calf_dyno_enclosure (Autodesk Fusion 360 design; units mm, degrees)
Autodesk Fusion 360 part; units mm, degrees
sketch "Outer shell blank profile" plane through (0, 0, 0) normal (0, 0, 1) x (1, 0, 0) in component "Base - print floor down"
  line L0 (10, 10) -> (100, 10)
  line L1 (100, 10) -> (100, 75)
  line L2 (100, 75) -> (10, 75)
  line L3 (10, 75) -> (10, 10)
  dimension "d23" = 10
  dimension "d24" = 10
  dimension "d25" = 90
  dimension "d26" = 65
  measures "d23" horizontal distance of origin L0.start
  measures "d24" vertical distance of origin L0.start
  measures "d25" horizontal distance of L0.start L0.end
  measures "d26" vertical distance of L0.end L1.end
extrude "Outer shell blank" add sketch "Outer shell blank profile" along normal blind 32 makes body 1 in component "Base - print floor down"
fillet "Rounded outside corners" radius 2 4 edges at (10, 75, 16) (100, 75, 16) (100, 10, 16) (10, 10, 16) on bodies 1 in component "Base - print floor down"
sketch "Electronics cavity profile" plane through (0, 0, 0) normal (0, 0, 1) x (1, 0, 0) in component "Base - print floor down"
  line L0 (12, 12) -> (98, 12)
  line L1 (98, 12) -> (98, 73)
  line L2 (98, 73) -> (12, 73)
  line L3 (12, 73) -> (12, 12)
  dimension "d32" = 12
  dimension "d33" = 12
  dimension "d34" = 86
  dimension "d35" = 61
  measures "d32" horizontal distance of origin L0.start
  measures "d33" vertical distance of origin L0.start
  measures "d34" horizontal distance of L0.start L0.end
  measures "d35" vertical distance of L0.end L1.end
extrude "Electronics cavity" cut sketch "Electronics cavity profile" along normal blind 31 from surface at 2 bodies 1 in component "Base - print floor down"
sketch "USB-C plug access profile" plane through (0, 0, 0) normal (0, 0, 1) x (1, 0, 0) in component "Base - print floor down"
  line L0 (9, 34.5) -> (13, 34.5)
  line L1 (13, 34.5) -> (13, 50.5)
  line L2 (13, 50.5) -> (9, 50.5)
  line L3 (9, 50.5) -> (9, 34.5)
  dimension "d39" = 9
  dimension "d40" = 34.5
  dimension "d41" = 4
  dimension "d42" = 16
  measures "d39" horizontal distance of origin L0.start
  measures "d40" vertical distance of origin L0.start
  measures "d41" horizontal distance of L0.start L0.end
  measures "d42" vertical distance of L0.end L1.end
extrude "USB-C plug access" cut sketch "USB-C plug access profile" along normal blind 10 from surface at 4 bodies 1 in component "Base - print floor down"
sketch "Drop-in load-cell cable notch profile" plane through (0, 0, 0) normal (0, 0, 1) x (1, 0, 0) in component "Base - print floor down"
  line L0 (97, 39) -> (101, 39)
  line L1 (101, 39) -> (101, 46)
  line L2 (101, 46) -> (97, 46)
  line L3 (97, 46) -> (97, 39)
  dimension "d46" = 97
  dimension "d47" = 39
  dimension "d48" = 4
  dimension "d49" = 7
  measures "d46" horizontal distance of origin L0.start
  measures "d47" vertical distance of origin L0.start
  measures "d48" horizontal distance of L0.start L0.end
  measures "d49" vertical distance of L0.end L1.end
extrude "Drop-in load-cell cable notch" cut sketch "Drop-in load-cell cable notch profile" along normal blind 8 from surface at 25 bodies 1 in component "Base - print floor down"
fillet "Rounded cable seat" radius 3.3 2 edges at (99, 39, 25) (99, 46, 25) on bodies 1 in component "Base - print floor down"
sketch "Snap window front outer_length * 0.23 profile" plane through (0, 0, 0) normal (0, 0, 1) x (1, 0, 0) in component "Base - print floor down"
  line L0 (26.4, 9) -> (35, 9)
  line L1 (35, 9) -> (35, 13)
  line L2 (35, 13) -> (26.4, 13)
  line L3 (26.4, 13) -> (26.4, 9)
  dimension "d55" = 26.4
  dimension "d56" = 9
  dimension "d57" = 8.6
  dimension "d58" = 4
  measures "d55" horizontal distance of origin L0.start
  measures "d56" vertical distance of origin L0.start
  measures "d57" horizontal distance of L0.start L0.end
  measures "d58" vertical distance of L0.end L1.end
extrude "Snap window front outer_length * 0.23" cut sketch "Snap window front outer_length * 0.23 profile" along normal blind 2.6 from surface at 17.7 bodies 1 in component "Base - print floor down"
sketch "Snap window back outer_length * 0.23 profile" plane through (0, 0, 0) normal (0, 0, 1) x (1, 0, 0) in component "Base - print floor down"
  line L0 (26.4, 72) -> (35, 72)
  line L1 (35, 72) -> (35, 76)
  line L2 (35, 76) -> (26.4, 76)
  line L3 (26.4, 76) -> (26.4, 72)
  dimension "d62" = 26.4
  dimension "d63" = 72
  dimension "d64" = 8.6
  dimension "d65" = 4
  measures "d62" horizontal distance of origin L0.start
  measures "d63" vertical distance of origin L0.start
  measures "d64" horizontal distance of L0.start L0.end
  measures "d65" vertical distance of L0.end L1.end
extrude "Snap window back outer_length * 0.23" cut sketch "Snap window back outer_length * 0.23 profile" along normal blind 2.6 from surface at 17.7 bodies 1 in component "Base - print floor down"
sketch "Snap window front outer_length * 0.77 profile" plane through (0, 0, 0) normal (0, 0, 1) x (1, 0, 0) in component "Base - print floor down"
  line L0 (75, 9) -> (83.6, 9)
  line L1 (83.6, 9) -> (83.6, 13)
  line L2 (83.6, 13) -> (75, 13)
  line L3 (75, 13) -> (75, 9)
  dimension "d69" = 75
  dimension "d70" = 9
  dimension "d71" = 8.6
  dimension "d72" = 4
  measures "d69" horizontal distance of origin L0.start
  measures "d70" vertical distance of origin L0.start
  measures "d71" horizontal distance of L0.start L0.end
  measures "d72" vertical distance of L0.end L1.end
extrude "Snap window front outer_length * 0.77" cut sketch "Snap window front outer_length * 0.77 profile" along normal blind 2.6 from surface at 17.7 bodies 1 in component "Base - print floor down"
sketch "Snap window back outer_length * 0.77 profile" plane through (0, 0, 0) normal (0, 0, 1) x (1, 0, 0) in component "Base - print floor down"
  line L0 (75, 72) -> (83.6, 72)
  line L1 (83.6, 72) -> (83.6, 76)
  line L2 (83.6, 76) -> (75, 76)
  line L3 (75, 76) -> (75, 72)
  dimension "d76" = 75
  dimension "d77" = 72
  dimension "d78" = 8.6
  dimension "d79" = 4
  measures "d76" horizontal distance of origin L0.start
  measures "d77" vertical distance of origin L0.start
  measures "d78" horizontal distance of L0.start L0.end
  measures "d79" vertical distance of L0.end L1.end
extrude "Snap window back outer_length * 0.77" cut sketch "Snap window back outer_length * 0.77 profile" along normal blind 2.6 from surface at 17.7 bodies 1 in component "Base - print floor down"
sketch "Cable tie anchor profile" plane through (0, 0, 0) normal (0, 0, 1) x (1, 0, 0) in component "Base - print floor down"
  line L0 (84, 37.5) -> (92, 37.5)
  line L1 (92, 37.5) -> (92, 47.5)
  line L2 (92, 47.5) -> (84, 47.5)
  line L3 (84, 47.5) -> (84, 37.5)
  dimension "d83" = 84
  dimension "d84" = 37.5
  dimension "d85" = 8
  dimension "d86" = 10
  measures "d83" horizontal distance of origin L0.start
  measures "d84" vertical distance of origin L0.start
  measures "d85" horizontal distance of L0.start L0.end
  measures "d86" vertical distance of L0.end L1.end
extrude "Cable tie anchor" add sketch "Cable tie anchor profile" along normal blind 5 from surface at 2 bodies 1 in component "Base - print floor down"
sketch "Cable tie tunnel profile" plane through (0, 0, 0) normal (0, 0, 1) x (1, 0, 0) in component "Base - print floor down"
  line L0 (83, 40.5) -> (93, 40.5)
  line L1 (93, 40.5) -> (93, 44.5)
  line L2 (93, 44.5) -> (83, 44.5)
  line L3 (83, 44.5) -> (83, 40.5)
  dimension "d90" = 83
  dimension "d91" = 40.5
  dimension "d92" = 10
  dimension "d93" = 4
  measures "d90" horizontal distance of origin L0.start
  measures "d91" vertical distance of origin L0.start
  measures "d92" horizontal distance of L0.start L0.end
  measures "d93" vertical distance of L0.end L1.end
extrude "Cable tie tunnel" cut sketch "Cable tie tunnel profile" along normal blind 2 from surface at 3 bodies 1 in component "Base - print floor down"
sketch "Lid plate profile" plane through (0, 0, 0) normal (0, 0, 1) x (1, 0, 0) in component "Lid - print outside face down"
  line L0 (10, 10) -> (100, 10)
  line L1 (100, 10) -> (100, 75)
  line L2 (100, 75) -> (10, 75)
  line L3 (10, 75) -> (10, 10)
  dimension "d97" = 10
  dimension "d98" = 10
  dimension "d99" = 90
  dimension "d100" = 65
  measures "d97" horizontal distance of origin L0.start
  measures "d98" vertical distance of origin L0.start
  measures "d99" horizontal distance of L0.start L0.end
  measures "d100" vertical distance of L0.end L1.end
extrude "Lid plate" add sketch "Lid plate profile" along normal blind 2 from surface at 32 separate body makes body 2 in component "Lid - print outside face down"
fillet "Lid outside corners" radius 2 4 edges at (10, 75, 33) (100, 75, 33) (100, 10, 33) (10, 10, 33) on bodies 2 in component "Lid - print outside face down"
sketch "Guide left front profile" plane through (0, 0, 0) normal (0, 0, 1) x (1, 0, 0) in component "Lid - print outside face down"
  line L0 (12.3, 12.3) -> (19.3, 12.3)
  line L1 (19.3, 12.3) -> (19.3, 13.5)
  line L2 (19.3, 13.5) -> (12.3, 13.5)
  line L3 (12.3, 13.5) -> (12.3, 12.3)
  dimension "d106" = 12.3
  dimension "d107" = 12.3
  dimension "d108" = 7
  dimension "d109" = 1.2
  measures "d106" horizontal distance of origin L0.start
  measures "d107" vertical distance of origin L0.start
  measures "d108" horizontal distance of L0.start L0.end
  measures "d109" vertical distance of L0.end L1.end
extrude "Guide left front" add sketch "Guide left front profile" along normal blind 3 from surface at 29 bodies 2 in component "Lid - print outside face down"
sketch "Guide left back profile" plane through (0, 0, 0) normal (0, 0, 1) x (1, 0, 0) in component "Lid - print outside face down"
  line L0 (12.3, 71.5) -> (19.3, 71.5)
  line L1 (19.3, 71.5) -> (19.3, 72.7)
  line L2 (19.3, 72.7) -> (12.3, 72.7)
  line L3 (12.3, 72.7) -> (12.3, 71.5)
  dimension "d113" = 12.3
  dimension "d114" = 71.5
  dimension "d115" = 7
  dimension "d116" = 1.2
  measures "d113" horizontal distance of origin L0.start
  measures "d114" vertical distance of origin L0.start
  measures "d115" horizontal distance of L0.start L0.end
  measures "d116" vertical distance of L0.end L1.end
extrude "Guide left back" add sketch "Guide left back profile" along normal blind 3 from surface at 29 bodies 2 in component "Lid - print outside face down"
sketch "Guide right front profile" plane through (0, 0, 0) normal (0, 0, 1) x (1, 0, 0) in component "Lid - print outside face down"
  line L0 (90.7, 12.3) -> (97.7, 12.3)
  line L1 (97.7, 12.3) -> (97.7, 13.5)
  line L2 (97.7, 13.5) -> (90.7, 13.5)
  line L3 (90.7, 13.5) -> (90.7, 12.3)
  dimension "d120" = 90.7
  dimension "d121" = 12.3
  dimension "d122" = 7
  dimension "d123" = 1.2
  measures "d120" horizontal distance of origin L0.start
  measures "d121" vertical distance of origin L0.start
  measures "d122" horizontal distance of L0.start L0.end
  measures "d123" vertical distance of L0.end L1.end
extrude "Guide right front" add sketch "Guide right front profile" along normal blind 3 from surface at 29 bodies 2 in component "Lid - print outside face down"
sketch "Guide right back profile" plane through (0, 0, 0) normal (0, 0, 1) x (1, 0, 0) in component "Lid - print outside face down"
  line L0 (90.7, 71.5) -> (97.7, 71.5)
  line L1 (97.7, 71.5) -> (97.7, 72.7)
  line L2 (97.7, 72.7) -> (90.7, 72.7)
  line L3 (90.7, 72.7) -> (90.7, 71.5)
  dimension "d127" = 90.7
  dimension "d128" = 71.5
  dimension "d129" = 7
  dimension "d130" = 1.2
  measures "d127" horizontal distance of origin L0.start
  measures "d128" vertical distance of origin L0.start
  measures "d129" horizontal distance of L0.start L0.end
  measures "d130" vertical distance of L0.end L1.end
extrude "Guide right back" add sketch "Guide right back profile" along normal blind 3 from surface at 29 bodies 2 in component "Lid - print outside face down"
sketch "End guide left front profile" plane through (0, 0, 0) normal (0, 0, 1) x (1, 0, 0) in component "Lid - print outside face down"
  line L0 (12.3, 12.3) -> (13.5, 12.3)
  line L1 (13.5, 12.3) -> (13.5, 19.3)
  line L2 (13.5, 19.3) -> (12.3, 19.3)
  line L3 (12.3, 19.3) -> (12.3, 12.3)
  dimension "d134" = 12.3
  dimension "d135" = 12.3
  dimension "d136" = 1.2
  dimension "d137" = 7
  measures "d134" horizontal distance of origin L0.start
  measures "d135" vertical distance of origin L0.start
  measures "d136" horizontal distance of L0.start L0.end
  measures "d137" vertical distance of L0.end L1.end
extrude "End guide left front" add sketch "End guide left front profile" along normal blind 3 from surface at 29 bodies 2 in component "Lid - print outside face down"
sketch "End guide left back profile" plane through (0, 0, 0) normal (0, 0, 1) x (1, 0, 0) in component "Lid - print outside face down"
  line L0 (12.3, 65.7) -> (13.5, 65.7)
  line L1 (13.5, 65.7) -> (13.5, 72.7)
  line L2 (13.5, 72.7) -> (12.3, 72.7)
  line L3 (12.3, 72.7) -> (12.3, 65.7)
  dimension "d141" = 12.3
  dimension "d142" = 65.7
  dimension "d143" = 1.2
  dimension "d144" = 7
  measures "d141" horizontal distance of origin L0.start
  measures "d142" vertical distance of origin L0.start
  measures "d143" horizontal distance of L0.start L0.end
  measures "d144" vertical distance of L0.end L1.end
extrude "End guide left back" add sketch "End guide left back profile" along normal blind 3 from surface at 29 bodies 2 in component "Lid - print outside face down"
sketch "End guide right front profile" plane through (0, 0, 0) normal (0, 0, 1) x (1, 0, 0) in component "Lid - print outside face down"
  line L0 (96.5, 12.3) -> (97.7, 12.3)
  line L1 (97.7, 12.3) -> (97.7, 19.3)
  line L2 (97.7, 19.3) -> (96.5, 19.3)
  line L3 (96.5, 19.3) -> (96.5, 12.3)
  dimension "d148" = 96.5
  dimension "d149" = 12.3
  dimension "d150" = 1.2
  dimension "d151" = 7
  measures "d148" horizontal distance of origin L0.start
  measures "d149" vertical distance of origin L0.start
  measures "d150" horizontal distance of L0.start L0.end
  measures "d151" vertical distance of L0.end L1.end
extrude "End guide right front" add sketch "End guide right front profile" along normal blind 3 from surface at 29 bodies 2 in component "Lid - print outside face down"
sketch "End guide right back profile" plane through (0, 0, 0) normal (0, 0, 1) x (1, 0, 0) in component "Lid - print outside face down"
  line L0 (96.5, 65.7) -> (97.7, 65.7)
  line L1 (97.7, 65.7) -> (97.7, 72.7)
  line L2 (97.7, 72.7) -> (96.5, 72.7)
  line L3 (96.5, 72.7) -> (96.5, 65.7)
  dimension "d155" = 96.5
  dimension "d156" = 65.7
  dimension "d157" = 1.2
  dimension "d158" = 7
  measures "d155" horizontal distance of origin L0.start
  measures "d156" vertical distance of origin L0.start
  measures "d157" horizontal distance of L0.start L0.end
  measures "d158" vertical distance of L0.end L1.end
extrude "End guide right back" add sketch "End guide right back profile" along normal blind 3 from surface at 29 bodies 2 in component "Lid - print outside face down"
sketch "Flexible snap front0 profile" plane through (0, 0, 0) normal (0, 0, 1) x (1, 0, 0) in component "Lid - print outside face down"
  line L0 (26.7, 12.3) -> (34.7, 12.3)
  line L1 (34.7, 12.3) -> (34.7, 13.5)
  line L2 (34.7, 13.5) -> (26.7, 13.5)
  line L3 (26.7, 13.5) -> (26.7, 12.3)
  dimension "d162" = 26.7
  dimension "d163" = 12.3
  dimension "d164" = 8
  dimension "d165" = 1.2
  measures "d162" horizontal distance of origin L0.start
  measures "d163" vertical distance of origin L0.start
  measures "d164" horizontal distance of L0.start L0.end
  measures "d165" vertical distance of L0.end L1.end
extrude "Flexible snap front0" add sketch "Flexible snap front0 profile" along normal blind 14 from surface at 18 bodies 2 in component "Lid - print outside face down"
sketch "Snap hook front0 profile" plane through (0, 0, 0) normal (0, 0, 1) x (1, 0, 0) in component "Lid - print outside face down"
  line L0 (26.7, 11.75) -> (34.7, 11.75)
  line L1 (34.7, 11.75) -> (34.7, 13.5)
  line L2 (34.7, 13.5) -> (26.7, 13.5)
  line L3 (26.7, 13.5) -> (26.7, 11.75)
  dimension "d169" = 26.7
  dimension "d170" = 11.75
  dimension "d171" = 8
  dimension "d172" = 1.75
  measures "d169" horizontal distance of origin L0.start
  measures "d170" vertical distance of origin L0.start
  measures "d171" horizontal distance of L0.start L0.end
  measures "d172" vertical distance of L0.end L1.end
extrude "Snap hook front0" add sketch "Snap hook front0 profile" along normal blind 2 from surface at 18 bodies 2 in component "Lid - print outside face down"
chamfer "Insertion ramp front0" distance 0.55 angle 45 1 edges at (30.7, 11.75, 18) on bodies 2 in component "Lid - print outside face down"
sketch "Flexible snap back0 profile" plane through (0, 0, 0) normal (0, 0, 1) x (1, 0, 0) in component "Lid - print outside face down"
  line L0 (26.7, 71.5) -> (34.7, 71.5)
  line L1 (34.7, 71.5) -> (34.7, 72.7)
  line L2 (34.7, 72.7) -> (26.7, 72.7)
  line L3 (26.7, 72.7) -> (26.7, 71.5)
  dimension "d177" = 26.7
  dimension "d178" = 71.5
  dimension "d179" = 8
  dimension "d180" = 1.2
  measures "d177" horizontal distance of origin L0.start
  measures "d178" vertical distance of origin L0.start
  measures "d179" horizontal distance of L0.start L0.end
  measures "d180" vertical distance of L0.end L1.end
extrude "Flexible snap back0" add sketch "Flexible snap back0 profile" along normal blind 14 from surface at 18 bodies 2 in component "Lid - print outside face down"
sketch "Snap hook back0 profile" plane through (0, 0, 0) normal (0, 0, 1) x (1, 0, 0) in component "Lid - print outside face down"
  line L0 (26.7, 71.5) -> (34.7, 71.5)
  line L1 (34.7, 71.5) -> (34.7, 73.25)
  line L2 (34.7, 73.25) -> (26.7, 73.25)
  line L3 (26.7, 73.25) -> (26.7, 71.5)
  dimension "d184" = 26.7
  dimension "d185" = 71.5
  dimension "d186" = 8
  dimension "d187" = 1.75
  measures "d184" horizontal distance of origin L0.start
  measures "d185" vertical distance of origin L0.start
  measures "d186" horizontal distance of L0.start L0.end
  measures "d187" vertical distance of L0.end L1.end
extrude "Snap hook back0" add sketch "Snap hook back0 profile" along normal blind 2 from surface at 18 bodies 2 in component "Lid - print outside face down"
chamfer "Insertion ramp back0" distance 0.55 angle 45 1 edges at (30.7, 73.25, 18) on bodies 2 in component "Lid - print outside face down"
sketch "Flexible snap front1 profile" plane through (0, 0, 0) normal (0, 0, 1) x (1, 0, 0) in component "Lid - print outside face down"
  line L0 (75.3, 12.3) -> (83.3, 12.3)
  line L1 (83.3, 12.3) -> (83.3, 13.5)
  line L2 (83.3, 13.5) -> (75.3, 13.5)
  line L3 (75.3, 13.5) -> (75.3, 12.3)
  dimension "d192" = 75.3
  dimension "d193" = 12.3
  dimension "d194" = 8
  dimension "d195" = 1.2
  measures "d192" horizontal distance of origin L0.start
  measures "d193" vertical distance of origin L0.start
  measures "d194" horizontal distance of L0.start L0.end
  measures "d195" vertical distance of L0.end L1.end
extrude "Flexible snap front1" add sketch "Flexible snap front1 profile" along normal blind 14 from surface at 18 bodies 2 in component "Lid - print outside face down"
sketch "Snap hook front1 profile" plane through (0, 0, 0) normal (0, 0, 1) x (1, 0, 0) in component "Lid - print outside face down"
  line L0 (75.3, 11.75) -> (83.3, 11.75)
  line L1 (83.3, 11.75) -> (83.3, 13.5)
  line L2 (83.3, 13.5) -> (75.3, 13.5)
  line L3 (75.3, 13.5) -> (75.3, 11.75)
  dimension "d199" = 75.3
  dimension "d200" = 11.75
  dimension "d201" = 8
  dimension "d202" = 1.75
  measures "d199" horizontal distance of origin L0.start
  measures "d200" vertical distance of origin L0.start
  measures "d201" horizontal distance of L0.start L0.end
  measures "d202" vertical distance of L0.end L1.end
extrude "Snap hook front1" add sketch "Snap hook front1 profile" along normal blind 2 from surface at 18 bodies 2 in component "Lid - print outside face down"
chamfer "Insertion ramp front1" distance 0.55 angle 45 1 edges at (79.3, 11.75, 18) on bodies 2 in component "Lid - print outside face down"
sketch "Flexible snap back1 profile" plane through (0, 0, 0) normal (0, 0, 1) x (1, 0, 0) in component "Lid - print outside face down"
  line L0 (75.3, 71.5) -> (83.3, 71.5)
  line L1 (83.3, 71.5) -> (83.3, 72.7)
  line L2 (83.3, 72.7) -> (75.3, 72.7)
  line L3 (75.3, 72.7) -> (75.3, 71.5)
  dimension "d207" = 75.3
  dimension "d208" = 71.5
  dimension "d209" = 8
  dimension "d210" = 1.2
  measures "d207" horizontal distance of origin L0.start
  measures "d208" vertical distance of origin L0.start
  measures "d209" horizontal distance of L0.start L0.end
  measures "d210" vertical distance of L0.end L1.end
extrude "Flexible snap back1" add sketch "Flexible snap back1 profile" along normal blind 14 from surface at 18 bodies 2 in component "Lid - print outside face down"
sketch "Snap hook back1 profile" plane through (0, 0, 0) normal (0, 0, 1) x (1, 0, 0) in component "Lid - print outside face down"
  line L0 (75.3, 71.5) -> (83.3, 71.5)
  line L1 (83.3, 71.5) -> (83.3, 73.25)
  line L2 (83.3, 73.25) -> (75.3, 73.25)
  line L3 (75.3, 73.25) -> (75.3, 71.5)
  dimension "d214" = 75.3
  dimension "d215" = 71.5
  dimension "d216" = 8
  dimension "d217" = 1.75
  measures "d214" horizontal distance of origin L0.start
  measures "d215" vertical distance of origin L0.start
  measures "d216" horizontal distance of L0.start L0.end
  measures "d217" vertical distance of L0.end L1.end
extrude "Snap hook back1" add sketch "Snap hook back1 profile" along normal blind 2 from surface at 18 bodies 2 in component "Lid - print outside face down"
chamfer "Insertion ramp back1" distance 0.55 angle 45 1 edges at (79.3, 73.25, 18) on bodies 2 in component "Lid - print outside face down"
fillet "Rounded snap roots" radius 0.8 4 edges at (79.3, 71.5, 32) (79.3, 13.5, 32) (30.7, 71.5, 32) (30.7, 13.5, 32) on bodies 2 in component "Lid - print outside face down"
component "Base - print floor down" placed x (1, 0, 0) y (0, 1, 0) z (0, 0, 1) at (0, 0, 0)
component "Lid - print outside face down" placed x (1, 0, 0) y (0, 1, 0) z (0, 0, 1) at (0, 0, 0)
equation "inside_length = 86 mm" comment "Clear cavity length"
equation "inside_width = 61 mm" comment "Clear cavity width"
equation "inside_height = 30 mm" comment "Floor to lid underside; clips occupy side margins"
equation "wall = 2 mm" comment "Wall thickness"
equation "floor_thickness = 2 mm" comment "Floor thickness"
equation "lid_thickness = 2 mm" comment "Lid plate"
equation "fit_clearance = 0.3 mm" comment "Per-side clearance of lid guides and clip stems"
equation "usb_width = 16 mm" comment "Opening for plug overmould"
equation "usb_height = 10 mm" comment "USB opening height"
equation "usb_bottom = 4 mm" comment "USB opening bottom above outside base bottom"
equation "cable_width = 7 mm" comment "Drop-in cable notch width"
equation "cable_depth = 7 mm" comment "Depth below lid seam"
equation "snap_length = 14 mm" comment "Flexible clip length"
equation "snap_thickness = 1.2 mm" comment "Flexible clip thickness"
equation "snap_width = 8 mm" comment "Clip width"
equation "snap_projection = 0.55 mm" comment "Hook projection beyond stem"
equation "hook_height = 2 mm" comment "Hook height"
equation "corner_radius = 2 mm" comment "Outside vertical corners"
equation "outer_length = inside_length + 2 * wall" comment "Derived exterior length"
equation "outer_width = inside_width + 2 * wall" comment "Derived exterior width"
equation "base_height = inside_height + floor_thickness" comment "Derived base height"
equation "usb_y = outer_width / 2" comment "USB opening lateral center"
equation "d25 = outer_length"
equation "d26 = outer_width"
equation "d28 = base_height"
equation "d31 = corner_radius"
equation "d32 = 10 mm + wall"
equation "d33 = 10 mm + wall"
equation "d34 = inside_length"
equation "d35 = inside_width"
equation "d36 = floor_thickness"
equation "d37 = inside_height + 1 mm"
equation "d40 = 10 mm + usb_y - usb_width / 2"
equation "d41 = wall + 2 mm"
equation "d42 = usb_width"
equation "d43 = usb_bottom"
equation "d44 = usb_height"
equation "d46 = 10 mm + outer_length - wall - 1 mm"
equation "d47 = 10 mm + outer_width / 2 - cable_width / 2"
equation "d48 = wall + 2 mm"
equation "d49 = cable_width"
equation "d50 = base_height - cable_depth"
equation "d51 = cable_depth + 1 mm"
equation "d54 = cable_width / 2 - 0.2 mm"
equation "d55 = 10 mm + outer_length * 0.23 - snap_width / 2 - fit_clearance"
equation "d57 = snap_width + 2 * fit_clearance"
equation "d58 = wall + 2 mm"
equation "d59 = base_height - snap_length - fit_clearance"
equation "d60 = hook_height + 2 * fit_clearance"
equation "d62 = 10 mm + outer_length * 0.23 - snap_width / 2 - fit_clearance"
equation "d63 = 10 mm + outer_width - wall - 1 mm"
equation "d64 = snap_width + 2 * fit_clearance"
equation "d65 = wall + 2 mm"
equation "d66 = base_height - snap_length - fit_clearance"
equation "d67 = hook_height + 2 * fit_clearance"
equation "d69 = 10 mm + outer_length * 0.77 - snap_width / 2 - fit_clearance"
equation "d71 = snap_width + 2 * fit_clearance"
equation "d72 = wall + 2 mm"
equation "d73 = base_height - snap_length - fit_clearance"
equation "d74 = hook_height + 2 * fit_clearance"
equation "d76 = 10 mm + outer_length * 0.77 - snap_width / 2 - fit_clearance"
equation "d77 = 10 mm + outer_width - wall - 1 mm"
equation "d78 = snap_width + 2 * fit_clearance"
equation "d79 = wall + 2 mm"
equation "d80 = base_height - snap_length - fit_clearance"
equation "d81 = hook_height + 2 * fit_clearance"
equation "d83 = 10 mm + outer_length - wall - 14 mm"
equation "d84 = 10 mm + outer_width / 2 - 5 mm"
equation "d87 = floor_thickness"
equation "d90 = 10 mm + outer_length - wall - 15 mm"
equation "d91 = 10 mm + outer_width / 2 - 2 mm"
equation "d94 = floor_thickness + 1 mm"
equation "d99 = outer_length"
equation "d100 = outer_width"
equation "d101 = base_height"
equation "d102 = lid_thickness"
equation "d105 = corner_radius"
equation "d106 = 10 mm + wall + fit_clearance"
equation "d107 = 10 mm + wall + fit_clearance"
equation "d110 = base_height - 3 mm"
equation "d113 = 10 mm + wall + fit_clearance"
equation "d114 = 10 mm + outer_width - wall - fit_clearance - 1.2 mm"
equation "d117 = base_height - 3 mm"
equation "d120 = 10 mm + outer_length - wall - fit_clearance - 7 mm"
equation "d121 = 10 mm + wall + fit_clearance"
equation "d124 = base_height - 3 mm"
equation "d127 = 10 mm + outer_length - wall - fit_clearance - 7 mm"
equation "d128 = 10 mm + outer_width - wall - fit_clearance - 1.2 mm"
equation "d131 = base_height - 3 mm"
equation "d134 = 10 mm + wall + fit_clearance"
equation "d135 = 10 mm + wall + fit_clearance"
equation "d138 = base_height - 3 mm"
equation "d141 = 10 mm + wall + fit_clearance"
equation "d142 = 10 mm + outer_width - wall - fit_clearance - 7 mm"
equation "d145 = base_height - 3 mm"
equation "d148 = 10 mm + outer_length - wall - fit_clearance - 1.2 mm"
equation "d149 = 10 mm + wall + fit_clearance"
equation "d152 = base_height - 3 mm"
equation "d155 = 10 mm + outer_length - wall - fit_clearance - 1.2 mm"
equation "d156 = 10 mm + outer_width - wall - fit_clearance - 7 mm"
equation "d159 = base_height - 3 mm"
equation "d162 = 10 mm + outer_length * 0.23 - snap_width / 2"
equation "d163 = 10 mm + wall + fit_clearance"
equation "d164 = snap_width"
equation "d165 = snap_thickness"
equation "d166 = base_height - snap_length"
equation "d167 = snap_length"
equation "d169 = 10 mm + outer_length * 0.23 - snap_width / 2"
equation "d170 = 10 mm + wall + fit_clearance - snap_projection"
equation "d171 = snap_width"
equation "d172 = snap_thickness + snap_projection"
equation "d173 = base_height - snap_length"
equation "d174 = hook_height"
equation "d176 = snap_projection"
equation "d177 = 10 mm + outer_length * 0.23 - snap_width / 2"
equation "d178 = 10 mm + outer_width - wall - fit_clearance - snap_thickness"
equation "d179 = snap_width"
equation "d180 = snap_thickness"
equation "d181 = base_height - snap_length"
equation "d182 = snap_length"
equation "d184 = 10 mm + outer_length * 0.23 - snap_width / 2"
equation "d185 = 10 mm + outer_width - wall - fit_clearance - snap_thickness"
equation "d186 = snap_width"
equation "d187 = snap_thickness + snap_projection"
equation "d188 = base_height - snap_length"
equation "d189 = hook_height"
equation "d191 = snap_projection"
equation "d192 = 10 mm + outer_length * 0.77 - snap_width / 2"
equation "d193 = 10 mm + wall + fit_clearance"
equation "d194 = snap_width"
equation "d195 = snap_thickness"
equation "d196 = base_height - snap_length"
equation "d197 = snap_length"
equation "d199 = 10 mm + outer_length * 0.77 - snap_width / 2"
equation "d200 = 10 mm + wall + fit_clearance - snap_projection"
equation "d201 = snap_width"
equation "d202 = snap_thickness + snap_projection"
equation "d203 = base_height - snap_length"
equation "d204 = hook_height"
equation "d206 = snap_projection"
equation "d207 = 10 mm + outer_length * 0.77 - snap_width / 2"
equation "d208 = 10 mm + outer_width - wall - fit_clearance - snap_thickness"
equation "d209 = snap_width"
equation "d210 = snap_thickness"
equation "d211 = base_height - snap_length"
equation "d212 = snap_length"
equation "d214 = 10 mm + outer_length * 0.77 - snap_width / 2"
equation "d215 = 10 mm + outer_width - wall - fit_clearance - snap_thickness"
equation "d216 = snap_width"
equation "d217 = snap_thickness + snap_projection"
equation "d218 = base_height - snap_length"
equation "d219 = hook_height"
equation "d221 = snap_projection"
named bodies: "Enclosure base", "Snap lid"
